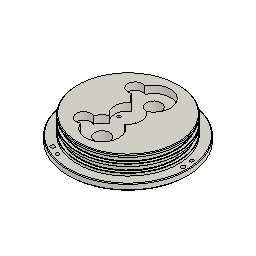
End_cap_drilling_charging (Autodesk Fusion 360 design; units mm, degrees)
Autodesk Fusion 360 part; units mm, degrees
sketch "Sketch1" plane through (0, 0, 0) normal (0, 1, 0) x (1, 0, 0)
  line L0 (0, 0) -> (45, 0)
  line L1 (45, 0) -> (45, -5)
  line L2 (45, -5) -> (38, -5)
  line L3 (38, -19) -> (0, -19)
  line L4 (0, -19) -> (0, 0)
  line L5 (38, -7) -> (35.7, -7)
  line L6 (35.7, -7) -> (35.7, -11)
  line L7 (35.7, -11) -> (38, -11)
  line L8 (38, -13) -> (35.7, -13)
  line L9 (35.7, -13) -> (35.7, -17)
  line L10 (35.7, -17) -> (38, -17)
  line L11 (38, -5) -> (38, -7)
  line L12 (38, -11) -> (38, -13)
  line L13 (38, -17) -> (38, -19)
  dimension "d2" = 45
  dimension "d4" = 5
  dimension "d5" = 7
  dimension "d9" = 4
  dimension "d10" = 4
  dimension "d11" = 2.3
  dimension "d13" = 2
  dimension "d14" = 2
  dimension "d15" = 2
  dimension "d16" = 19
  constraint coincident L0.start L4.end
  constraint horizontal L0
  constraint perpendicular L0 L1
  constraint perpendicular L1 L2
  constraint perpendicular L2 L11
  constraint perpendicular L1 L3
  constraint perpendicular L0 L4
  constraint perpendicular L5 L11
  constraint perpendicular L5 L6
  constraint perpendicular L7 L11
  constraint coincident L8.start L11
  constraint perpendicular L8 L11
  constraint perpendicular L8 L9
  constraint coincident L10.end L11
  constraint perpendicular L10 L11
  constraint collinear L11 L12
  constraint coincident L7.end L11
  constraint collinear L6 L9
  constraint collinear L12 L13
  measures "d2" distance of L0.start L0.end
  measures "d4" distance of L0.end L1.end
  measures "d5" distance of L1.end L2.end
  measures "d9" distance of L5.end L6.end
  measures "d10" distance of L8.end L9.end
  measures "d11" distance of L8.start L8.end
  measures "d13" distance of L3.start L10.end
  measures "d14" distance of L7.end L8.start
  measures "d15" distance of L2.end L5.start
  measures "d16" distance of L3.end L0.start
revolve "Revolve1" add sketch "Sketch1" angle 360 about axis through (0, 0, 19) along (0, 0, -1)
chamfer "Chamfer1" distance 1 angle 45 1 edges at (-41.9547, -16.2727, 0)
chamfer "Chamfer2" distance 0.5 angle 45 1 edges at (-35.4284, -13.7414, 19)
fillet "Fillet1" radius 0.2 4 edges at (-35.4284, -13.7414, 17) (-35.4284, -13.7414, 13) (-35.4284, -13.7414, 11) (-35.4284, -13.7414, 7)
fillet "Fillet2" radius 0.3 2 faces at (35.5226, -3.5546, 15.6667) (35.6556, -1.7795, 8.3333)
sketch "Sketch3" plane through (0, 0, 0) normal (0, 0, -1) x (1, 0, 0)
  circle A0 centre (0, 0) radius 44
  point P0 (41.5, 0)
  point P1 (40.8695, -7.2064)
  dimension "d50" = 41.5
  dimension "d51" = 41.5
  dimension "d52" = 10
  constraint horizontal A0.centre P0
  measures "d50" distance of A0.centre P0
  measures "d51" distance of A0.centre P1
  measures "d52" angle of A0.centre P0 P1
hole "Hole4" at (40.8695, 7.2064, 0) direction (0, 0, 1) diameter 2.529 end through all
thread "Thread3" "ISO Metric profile 3.0 M3x0.5 6H" thread offset 0 thread depth 10
hole "Hole5" at (41.5, 0, 0) direction (0, 0, 1) diameter 3 end through all
pattern_circular "C-Pattern6" count 3 over 360 about axis through (0, 0, 1.75) along (0, 0, 1) of "Hole4", "Hole5"
chamfer "Chamfer3" distance 0.5 angle 45 1 edges at (-41.9547, -16.2727, 5)
sketch "Sketch4" plane through (0, 0, 0) normal (0, 0, 1) x (1, 0, 0)
  circle A0 centre (0, -19.4) radius 5.6
  line L0 (0, 0) -> (0, 18.1147) construction
  circle A1 centre (0, -19.4) radius 7
  circle A2 centre (0, -19.4) radius 12.5
  circle A3 centre (0, -19.4) radius 9.5
  circle A4 centre (0, 0) radius 35.7
  line L1 (0, 0) -> (-34.5804, 0) construction
  circle A5 centre (0, 0) radius 19.4
  circle A6 centre (0, 19.4) radius 12.5
  circle A7 centre (0, 19.4) radius 9.5
  circle A8 centre (0, 19.4) radius 7
  circle A9 centre (0, 19.4) radius 5.6
  circle A10 centre (0, 0) radius 10
  line L2 (0, 19.4) -> (-2.8543, 3.6567)
  circle A11 centre (-14, -19.4) radius 5.5
  circle A12 centre (-14, 19.4) radius 5.5
  line L3 (0, -19.4) -> (-18, -19.4) construction
  dimension "d62" = 11.2
  dimension "d63" = 14
  dimension "d65" = 25
  dimension "d75" = 19
  dimension "d108" = 38.8
  dimension "d147" = 20
  dimension "d149" = 16
  dimension "d159" = 11
  dimension "d160" = 18
  dimension "d161" = 19.4
  dimension "d162" = 14
  constraint coincident L0.start A4.centre
  constraint vertical L0
  constraint concentric A0 A1
  constraint concentric A1 A2
  constraint concentric A1 A3
  constraint coincident A0.centre A5
  constraint coincident A5 A6.centre
  constraint concentric A6 A7
  constraint equal A2 A6
  constraint equal A3 A7
  constraint concentric A6 A8
  constraint concentric A6 A9
  constraint equal A1 A8
  constraint equal A0 A9
  constraint horizontal L1
  constraint coincident A6.centre A7.centre
  constraint coincident L0 A6.centre
  constraint coincident A0.centre L0
  constraint symmetric L1 A11 A12
  constraint coincident A0.centre A1.centre
  constraint coincident A11.centre L3
  measures "d62" diameter of A0
  measures "d63" diameter of A1
  measures "d65" diameter of A2
  measures "d75" diameter of A3
  measures "d108" diameter of A5
  measures "d147" diameter of A10
  measures "d149" distance of A6.centre L2.end
  measures "d159" diameter of A11
  measures "d160" distance of A0.centre L3.end
  measures "d161" vertical distance of L0.start A11.centre
  measures "d162" horizontal distance of L0.start A11.centre
extrude "Extrude1" cut sketch "Sketch4" along normal through all contours A0 A5 | A0 A5 | A5 A9 L2 | A5 A9 | A5 A9 L2
extrude "Extrude3" cut sketch "Sketch4" along normal blind 19 and the other way blind -13.5 contours A0 A5 | A0 A1 A5 | A0 A5 | A0 A1 A5 | A1 A3 A5 A11 | A1 A3 A5 A10 A11 | A2 A3 A5 A11 | A2 A3 A5 A10 | A3 A5 A11 | A3 A5 A11 | A3 A10 | A2 A3 A10 | A2 A3 A5 A11 | A2 A3 A5 A11 | A2 A3 A10 A11 | A2 A6 A10 | A2 A5 A11 | A2 A5 A11 | A5 A6 A7 A10 | A5 A6 A7 A12 | A6 A10 L2 | A6 A7 A10 L2 A12 | A6 A7 A10 L2 | A5 A7 A8 A10 L2 | A5 A7 A8 A12 | A5 A6 A12 | A5 A6 A12 | A5 A6 A7 A12 | A7 A10 L2 | A7 A10 | A5 A8 A9 L2 | A5 A8 A9 | A5 A6 A7 A12 | A5 A7 A8 L2 A12 | A5 A7 A12 | A5 A9 L2 | A5 A9 | A5 A8 A9 L2 | A5 A7 A12 | A5 A9 L2
extrude "Extrude4" cut sketch "Sketch4" along normal blind 1.5 contours A0 A1 A5 | A0 A1 A5 | A5 A8 A9 L2 | A5 A8 A9 | A5 A8 A9 L2
ref_plane "Arbeitsebene2" through (0, 0, 19) normal (0, 0, 1) x (1, 0, 0)
sketch "Skizze12" plane through (0, 0, 13.5) normal (0, 0, 1) x (1, 0, 0)
  circle A0 centre (0, 19.4) radius 5.6
  circle A1 centre (0, -19.4) radius 5.6
  arc A2 (-11.5, 14.501) -> (-5.651, 8.2503) centre (0, 19.4) ccw
  line L0 (-9.5, -3) -> (-9.5, 3)
  line L1 (-1.15, 5.75) -> (1.15, 5.75)
  line L2 (1.15, 5.75) -> (1.15, -5.75)
  line L3 (1.15, -5.75) -> (-1.15, -5.75)
  line L4 (-1.15, -5.75) -> (-1.15, 5.75)
  line L5 (-1.15, 5.75) -> (1.15, -5.75) construction
  line L6 (1.15, 5.75) -> (-1.15, -5.75) construction
  line L7 (3.5, 3) -> (3.5, -3)
  line L8 (-9.5, 3) -> (3.5, 3)
  line L9 (3.5, -3) -> (-9.5, -3)
  arc A3 (5.651, -8.2503) -> (5.651, 8.2503) centre (0, 0) ccw
  arc A4 (-5.651, 8.2503) -> (-5.651, -8.2503) centre (0, 0) ccw
  arc A5 (-5.651, -8.2503) -> (-11.5, -14.501) centre (0, -19.4) ccw
  arc A6 (-11.5, -14.501) -> (-11.5, -24.299) centre (-14, -19.4) ccw
  arc A7 (-11.5, -24.299) -> (5.651, -8.2503) centre (0, -19.4) ccw
  arc A8 (5.651, 8.2503) -> (-11.5, 24.299) centre (0, 19.4) ccw
  arc A9 (-11.5, 24.299) -> (-11.5, 14.501) centre (-14, 19.4) ccw
  point P0 (-6.8, 0)
  point P1 (6, 0)
  dimension "d139" = 2.3
  dimension "d140" = 11.5
  dimension "d142" = 3.5
  dimension "d143" = 3
  dimension "d144" = 6
  dimension "d145" = 13
  dimension "d151" = 6
  constraint horizontal L8
  constraint horizontal L1
  constraint perpendicular L1 L2
  constraint parallel L1 L3
  constraint parallel L2 L4
  constraint coincident L5 A3.centre
  constraint coincident L6 A3.centre
  constraint coincident A3.centre A4.centre
  constraint perpendicular L7 L8
  constraint horizontal P1 A3.centre
  measures "d139" distance of L1.start L1.end
  measures "d140" distance of L1.start L3.end
  measures "d142" distance of A3.centre L7
  measures "d143" distance of A3.centre L8
  measures "d144" distance of L8 L9
  measures "d145" distance of L0 L7
  measures "d151" horizontal distance of P1 A3.centre
hole "Bohrung7" at (-6.8, 0, 13.5) direction (0, 0, -1) diameter 2.529 depth 7 tip angle 118
thread "Gewinde5" "ISO Metric profile 3.0 M3x0.5 6H" major diameter 3.086 minor diameter 2.529 pitch 0.5 angle 60 resizes the face on face at (-6.6741, -1.2582, 11.1667) from (-6.8, 0, 13.5) to (-6.8, 0, 7.5)
hole "Bohrung8" at (6, 0, 13.5) direction (0, 0, -1) diameter 6.5 depth 7.05 tip angle 118
extrude "Extrusion9" [suppressed]
equation "D_i = 76 mm" comment "Inner Diameter of Cylinder"
equation "d2 = ( D_i + 2 * t ) / 2"
equation "t = 7 mm" comment "Thickness of cylinder wall"
equation "d5 = t"
equation "Oring_depth = 2.3 mm" comment "Depth of Oring Groove"
equation "Oring_width = 4 mm" comment "Width of Oring Groove"
equation "d9 = Oring_width"
equation "d10 = Oring_width"
equation "d11 = Oring_depth"
equation "d50 = D_i / 2 + t / 2"
equation "d51 = d50"
equation "d71 = -19 mm + 5.5 mm"
equation "d108 = 19.4 * 2 mm"
equation "d161 = ( 38.8 / 2 ) * 1 mm"
